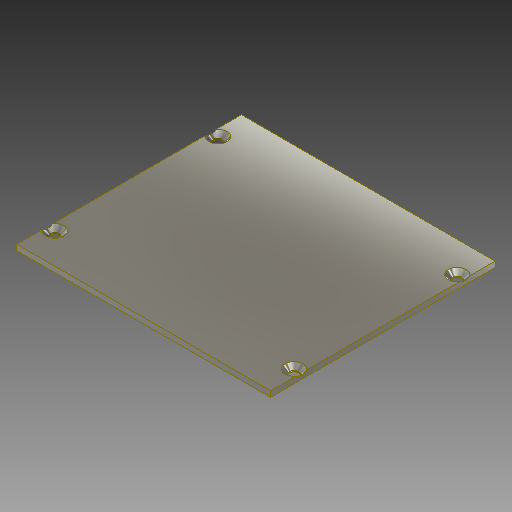
# Autodesk Inventor part: blech_2mm
Saved by Autodesk Inventor 2017 (Build 210142000, 142)
## iProperties
Part Number: blech_2mm
Material: Generisch
Document SubType Name: Modeling
Designer: Philomena-Theresa
Density: 1 g/cm^3
Appearance: Vorgabe
Author: Philomena-Theresa
Autodesk Inventor part; units mm, degrees
ref_plane "YZ Plane" through (0, 0, 0) normal (1, 0, 0) x (0, 1, 0)
ref_plane "XZ Plane" through (0, 0, 0) normal (0, 1, 0) x (-1, 0, 0)
ref_plane "XY Plane" through (0, 0, 0) normal (0, 0, 1) x (1, 0, 0)
sketch "Skizze1" plane through (0, 0, 0) normal (0, 0, 1) x (1, 0, 0)
  line L0 (0, 0) -> (90.4, 0)
  line L1 (90.4, 0) -> (90.4, 80)
  line L2 (90.4, 80) -> (0, 80)
  line L3 (0, 80) -> (0, 0)
  line L4 (2.6, 69.1) -> (87.8, 69.1) construction
  line L5 (87.8, 69.1) -> (87.8, 10.9) construction
  circle A0 centre (2.6, 69.1) radius 1.6
  circle A1 centre (2.6, 10.9) radius 1.6
  circle A2 centre (87.8, 69.1) radius 1.6
  circle A3 centre (87.8, 10.9) radius 1.6
  line L6 (65.2, 69.1) -> (82.75, 69.1) construction
  line L7 (25.2, 69.1) -> (42.75, 69.1) construction
  dimension "d0" = 90.4
  dimension "d1" = 80
  dimension "d5" = 87.8
  dimension "d6" = 3.2
  constraints: 16 end point, 4 centre point, 4 horizontal, 3 coincident, 3 equal radius, 2 parallel, 2 perpendicular, 1 collinear
  measures "d0" distance of L0.start L0.end
  measures "d1" distance of L0.end L1.end
  measures "d5" distance from line of L0.start L5
  measures "d6" diameter of A0
extrude "Extrusion1" add sketch "Skizze1" along normal blind 2
chamfer "Fase1" distance 1.6 angle 45 4 edges at (86.2, 10.9, 2) (1, 10.9, 2) (1, 69.1, 2) (86.2, 69.1, 2)
